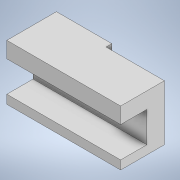
# Autodesk Inventor part: Practica 6
Saved by Autodesk Inventor 2020.2 (Build 242310000, 310)
## iProperties
Created: 2020-02-16
Part Number: Practica 6
Material: Genérico
Document SubType Name: Modeling
Designer: Luis Gallardo
Density: 1 g/cm^3
Appearance: Valor por defecto
Author: Luis Gallardo
Autodesk Inventor part; units mm, degrees
ref_plane "YZ Plane" through (0, 0, 0) normal (1, 0, 0) x (0, 1, 0)
ref_plane "XZ Plane" through (0, 0, 0) normal (0, 1, 0) x (-1, 0, 0)
ref_plane "XY Plane" through (0, 0, 0) normal (0, 0, 1) x (1, 0, 0)
sketch "Boceto2" plane through (0, 0, 0) normal (0, 1, 0) x (-1, 0, 0)
  line L0 (0, 0) -> (-78, 0)
  line L1 (-78, 0) -> (-78, -30)
  line L2 (-78, -30) -> (-38, -30)
  line L3 (-38, -30) -> (-38, -36)
  line L4 (-38, -36) -> (0, -36)
  line L5 (0, -36) -> (0, 0)
  dimension "d2" = 78
  dimension "d3" = 36
  dimension "d4" = 30
  dimension "d5" = 38
  constraints: 12 end point, 5 perpendicular, 1 horizontal
  measures "d2" distance of L0.start L0.end
  measures "d3" distance between parallel lines of L4 L0
  measures "d4" distance between parallel lines of L2 L0
  measures "d5" distance between parallel lines of L3 L5
extrude "Extrusión1" add sketch "Boceto2" along normal blind 38
sketch "Boceto3" plane through (0, 0, -36) normal (-1, 0, 0) x (0, 0, 1)
  line L0 (0, 0) -> (36, 0) construction
  line L1 (36, 0) -> (36, 6) construction
  line L2 (36, 0) -> (36, 38) construction
  line L3 (36, 6) -> (36, 27) construction
  line L4 (36, 27) -> (36, 38) construction
  line L5 (36, 6) -> (18, 6)
  line L6 (18, 6) -> (18, 27)
  line L7 (18, 27) -> (36, 27)
  line L8 (36, 6) -> (36, 27)
  dimension "d8" = 6
  dimension "d9" = 21
  dimension "d10" = 38
  dimension "d11" = 18
  constraints: 14 end point, 3 perpendicular, 2 collinear, 2 point on line
  measures "d8" distance of L0.end L1.end
  measures "d9" distance of L1.end L3.end
  measures "d10" distance of L0.end L2.end
  measures "d11" distance of L1.end L5.end
extrude "Extrusión2" cut sketch "Boceto3" against normal through all
sketch "Boceto4" plane through (38, 0, -36) normal (0, 0, -1) x (-1, 0, 0)
  line L0 (38, 27) -> (38, 38) construction
  line L1 (38, 38) -> (38, 19) construction
  line L2 (38, 19) -> (19, 19) construction
  line L3 (0, 0) -> (0, 38) construction
  circle A0 centre (19, 19) radius 8
  point P0 (38, 0)
  dimension "d14" = 19
  dimension "d15" = 19
  dimension "d16" = 16
  constraints: 4 end point, 1 centre point, 1 coincident, 1 collinear, 1 perpendicular
  measures "d14" distance of L0.end L1.end
  measures "d15" distance of L1.end L2.end
  measures "d16" diameter of A0
extrude "Extrusión3" cut sketch "Boceto4" against normal through all
chamfer "Chaflán1" distance 2 angle 45 4 edges at (19, 38, -36) (0, 19, -36) (19, 0, -36) (38, 19, -36)
